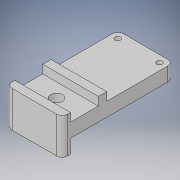
# Autodesk Inventor part: PinionHolder
Saved by Autodesk Inventor 2019 (Build 230136000, 136)
## iProperties
Created: 2019-08-06
Part Number: PinionHolder
Material: Generic
Document SubType Name: Modeling
Designer: aorfi
Density: 1 g/cm^3
Appearance: Default
Author: aorfi
Autodesk Inventor part; units mm, degrees
ref_plane "YZ Plane" through (0, 0, 0) normal (1, 0, 0) x (0, 1, 0)
ref_plane "XZ Plane" through (0, 0, 0) normal (0, 1, 0) x (-1, 0, 0)
ref_plane "XY Plane" through (0, 0, 0) normal (0, 0, 1) x (1, 0, 0)
sketch "Sketch1" plane through (0, 0, 0) normal (0, 1, 0) x (-1, 0, 0)
  line L0 (10, 20) -> (-10, 20)
  line L1 (-10, 20) -> (-10, -20)
  line L2 (-10, -20) -> (10, -20)
  line L3 (10, -20) -> (10, 20)
  line L4 (10, 20) -> (-10, -20) construction
  line L5 (-10, 20) -> (10, -20) construction
  point P0 (0, 0)
  dimension "d2" = 20
  dimension "d3" = 40
  constraints: 12 end point, 2 midpoint, 2 parallel, 1 horizontal, 1 perpendicular
  measures "d2" distance of L1.end L2.end
  measures "d3" distance of L0.end L1.end
extrude "Extrusion1" add sketch "Sketch1" along normal mid plane 5
sketch "Sketch2" plane through (0, 2.5, 0) normal (0, 1, 0) x (1, 0, 0)
  line L0 (10, -4) -> (-10, -4)
  line L1 (-10, -4) -> (-10, -7)
  line L2 (-10, -7) -> (10, -7)
  line L3 (10, -7) -> (10, -4)
  line L4 (10, -17) -> (-10, -17)
  line L5 (-10, -17) -> (-10, -20)
  line L6 (-10, -20) -> (10, -20)
  line L7 (10, -20) -> (10, -17)
  line L8 (10, -20) -> (10, 20) projected
  line L9 (-10, 20) -> (-10, -20) projected
  line L10 (10, 20) -> (-10, 20) projected
  line L11 (-10, -20) -> (10, -20) projected
  point P0 (0, 0)
  dimension "d4" = 3
  dimension "d5" = 3
  dimension "d6" = 10
  constraints: 16 end point, 5 collinear, 4 parallel, 2 horizontal, 2 perpendicular
  measures "d4" distance of L2.end L0.start
  measures "d5" distance of L6.end L4.start
  measures "d6" distance between parallel lines of L4 L2
extrude "Extrusion2" add sketch "Sketch2" along normal blind 3 contours L3 L2 L1 L0 | L7 L6 L5 L4
sketch "Sketch3" plane through (0, 2.5, 0) normal (0, 1, 0) x (1, 0, 0)
  line L0 (10, -7) -> (-10, -7) projected
  line L1 (-10, -7) -> (-10, -17) projected
  line L2 (-10, -17) -> (10, -17) projected
  line L3 (10, -17) -> (10, -7) projected
  line L4 (10, -17) -> (-10, -17) projected
  point P0 (0, 0)
  point P1 (0, -12)
  point P2 (-10, -12)
  point P3 (0, -17)
  constraints: 2 midpoint, 1 horizontal alignment, 1 vertical alignment
hole "Hole1" at (0, 2.5, 12) direction (0, -1, 0) diameter 4.305 end through all clearance for "Flat Head Machine Screw (82)" size "#6" standard "Ansi Unified Screw Threads"
sketch "Sketch4" plane through (0, -2.5, 0) normal (0, -1, 0) x (1, 0, 0)
  circle A0 centre (0, -4.677) radius 3.9688
  circle A1 centre (0, 12) radius 2.1525 projected
  point P0 (0, 0)
  dimension "d16" = 7.9375
  dimension "d17" = 16.677
  constraints: 1 centre point, 1 vertical alignment
  measures "d16" diameter of A0
  measures "d17" distance of A0.centre A1.centre
extrude "Extrusion3" add sketch "Sketch4" along normal blind 4 contours A0
sketch "Sketch6" plane through (0, -2.5, 0) normal (0, -1, 0) x (1, 0, 0)
  circle A0 centre (7.5, -17.5) radius 1
  circle A1 centre (-7.5, -17.5) radius 1
  line L0 (-10, -20) -> (10, -20) projected
  line L1 (10, -20) -> (10, 20) projected
  line L2 (-10, 20) -> (-10, -20) projected
  point P0 (0, 0)
  point P1 (-8, -17.5)
  point P2 (8, -17.5)
  point P3 (10, -15.5)
  point P4 (10, 15.5)
  point P5 (-10, 15.5)
  point P6 (-10, -15.5)
  dimension "d28" = 2
  dimension "d29" = 2
  dimension "d30" = 2.5
  dimension "d31" = 2.5
  dimension "d32" = 2.5
  constraints: 2 centre point, 1 horizontal alignment, 1 other
  measures "d28" diameter of A0
  measures "d29" diameter of A1
  measures "d31" distance from line of L1 A0.centre
  measures "d32" distance from line of L2 A1.centre
extrude "Extrusion5" cut sketch "Sketch6" against normal through all
sketch "Sketch8" plane through (0, -2.5, 0) normal (0, -1, 0) x (1, 0, 0)
  line L0 (10, 20) -> (10, 17) projected
  line L1 (10, 17) -> (-10, 17) projected
  line L2 (10, 20) -> (-10, 20)
  line L3 (-10, 20) -> (-10, 17)
  line L4 (-10, 17) -> (10, 17)
  line L5 (10, 17) -> (10, 20)
  point P0 (0, 0)
  constraints: 8 end point, 2 parallel, 1 horizontal, 1 perpendicular
extrude "Extrusion6" add sketch "Sketch8" along normal blind 5
sketch "Sketch9" plane through (0, -7.5, 0) normal (0, -1, 0) x (1, 0, 0)
  circle A0 centre (8, 18.5) radius 1
  circle A1 centre (-8, 18.5) radius 1
  line L0 (10, 17) -> (10, 20) projected
  line L1 (10, 20) -> (-10, 20) projected
  line L2 (-10, 20) -> (-10, 17) projected
  point P0 (0, 0)
  dimension "d38" = 2
  dimension "d39" = 2
  dimension "d40" = 2
  dimension "d41" = 1.5
  dimension "d42" = 2
  constraints: 2 centre point, 1 horizontal alignment
  measures "d38" diameter of A0
  measures "d39" diameter of A1
  measures "d40" distance from line of L0 A0.centre
  measures "d41" distance from line of L1 A0.centre
  measures "d42" distance from line of L2 A1.centre
extrude "Extrusion7" cut sketch "Sketch9" against normal blind 3
fillet "Fillet2" radius 2 4 edges at (-10, -1, 20) (-10, 0, -20) (10, 0, -20) (10, -1, 20)
equation "\"d5\" = d4"
equation "\"d31\" = d30"
equation "\"d32\" = d30"
equation "\"d42\" = d40"
body "Solid1"
